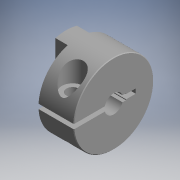
# Autodesk Inventor part: MCOCWK26-6_c
Saved by Autodesk Inventor 2017.3 (Build 213256000, 256)
## iProperties
Part Number: MCOCWK26-6_c
Material: Generic
Catalog Web Link: www.cadenas.de
Description: MCOC_coup-Couplings - Oldham Clamping Type
Vendor: MISUMI
Document SubType Name: Modeling
Designer: partserver
Manufacturer: MISUMI
Mass: 5.59398 g
Surface Area: 28.1267 cm^2
Volume: 5.59398 cm^3
Density: 1 g/cm^3
Appearance: PSOLRGB-192-192-192
Category: PARTsolutions
Company: MISUMI
Title: MCOCWK26-6
Author: Cadenas PARTsolutions
Comments: Couplings - Oldham Clamping Type
PSOL_IDENT_0: {$CADENAS_DATA\23d-libs\misumi\metric\50_couplings\mcoc\mcoc_coup.prj},208 {VTYP=3D},{NB=MCOCWK26-6_
PSOL_IDENT_1: c},{LINA=MCOCWK26-6},{NN=MCOC_coup},{DATE=30.03.2018 07:24:20},{GEOMDATE=05.12.2013 00:00:00},{VERSI
PSOL_IDENT_2: ON=},{LINEID=30},{WBVAR=HS,KGHS,ALT1,LDC,ALT2,RDC,DD,KGWC},{WBNUMERIC=LDC,RDC,DD}  {NB=MCOCWK26-6_c}
PSOL_IDENT_3: ,{LINA=MCOCWK26-6},{KT=DUMMY},{PN=MCOCWK26-6},{HS=},{KGHS=MCOCWK},{KGHSALG='MCOCLK','d1 (One Side)','
PSOL_IDENT_4: MCOCRK','d2 (One Side)','MCOCWK','d1*d2 (Both Sides)'},{MATH=304 Stainless Steel Sintered Alloy},{MA
PSOL_IDENT_5: TS=Carbon Reinforced Resin},{AC=Hexagon Socket Head Cap Screw},{TYPE=MCOCWK},{NO=26},{ALT1=},{ALT1AL
PSOL_IDENT_6: G=},{ALT13D=6},{DLALT1=6},{LDC=0.00},{LDCMIN=6},{LDCALG=0},{ALT2=},{ALT2ALG=},{ALT2ALG1= '', 'w/o RD
PSOL_IDENT_7: C (Shaft Hole Diameter Right Shaft)','RDC','with RDC (Shaft Hole Diameter Right Shaft)'},{ALT23D=6},
PSOL_IDENT_8: {RDC=0.00},{RDCALG=[0]},{DD=6.00},{DDALG=6,6.35,7,8,9.53,10,11,12},{DDPN=-6},{D=26.0},{D1=27},{D2=29
PSOL_IDENT_9: },{DD3=12.0},{L=30.4},{LL=11.5},{A=8.4},{F=5.0},{M=M4},{T=3.0},{ALTALG2='','Select RDC'},{HSALG='MCO
PSOL_IDENT_10: C','Standard Hole','','Key Groove Hole'},{TSIMD=4},{R1=7},{SC1=5.000},{SC2=5.000},{B=5.400},{L9=1.20
PSOL_IDENT_11: 0},{W=7.000},{G=4.000},{TT=1},{BB=2},{HSX=MCOCXK},{Z=7.155},{Z1=1.500},{KGWC=},{KGWCALG= '' , 'N/A'
PSOL_IDENT_12: },{KGWCPN=},{KGWC1=0},{TTKGW=0.0},{CIF=1},{BL=12}
NB: MCOCWK26-6_c
NN: MCOC_coup
NT: Couplings - Oldham Clamping Type
NBSYN: $PN._c
LINA: MCOCWK26-6
CATALOG: Misumi
PN: MCOCWK26-6
HS: Key Groove Hole
KGHS: d1*d2 (Both Sides)
NO: 26
ALT1: w/o LDC (Shaft Hole Diameter Left Shaft)
LDC: 0
ALT2: w/o RDC (Shaft Hole Diameter Right Shaft)
RDC: 0
DD: 6
D: 26
D1: 27
D2: 29
DD3: 12
L: 30.4
LL: 11.5
A: 8.4
F: 5
M: M4
T: 3.0
KGWC: N/A
SUPPLIER: MISUMI
ARTICLENO: MCOCWK26-6_c
BOMINFO: MCOCWK26-6
CREATOR: CADENAS GmbH
Autodesk Inventor part; units mm, degrees
sketch "Sketch_1" plane through (0, 0, 0) normal (0, 0, 1) x (1, 0, 0)
  line L0 (15.5, 0) -> (0, 0)
  line L1 (0, 0) -> (0, 12.8)
  line L2 (0, 12.8) -> (0.2, 13)
  line L3 (0.2, 13) -> (15.5, 13)
  line L4 (15.5, 13) -> (15.5, 0)
  line L5 (15.5, 0) -> (0, 0)
  constraints: 12 end point
revolve "Revolution1" add sketch "Sketch_1" angle 360 about axis through (15.5, 0, 0) along (1, 0, 0)
sketch "Sketch_6" plane through (0, 0, 0) normal (1, 0, 0) x (0, 1, 0)
  line L0 (-13, 0.75) -> (-13, -0.75)
  line L1 (-13, -0.75) -> (0, -0.75)
  line L2 (0, -0.75) -> (0, 0.75)
  line L3 (0, 0.75) -> (-13, 0.75)
  constraints: 8 end point
extrude "Extrusion1" cut sketch "Sketch_6" along normal blind 11.5
sketch "Sketch_7" plane through (5, 0, 0) normal (1, 0, 0) x (0, 0, -1)
  line L0 (-13, -8.4) -> (13, -8.4)
  line L1 (13, -8.4) -> (13, -11.9)
  line L2 (13, -11.9) -> (5, -11.9)
  line L3 (5, -11.9) -> (5, -10.4)
  line L4 (5, -10.4) -> (0.75, -10.4)
  line L5 (0.75, -10.4) -> (0.75, -8.4)
  line L6 (0.75, -8.4) -> (13, -8.4)
  constraints: 14 end point
revolve "Revolution2" cut sketch "Sketch_7" angle 360 about axis through (5, -8.4, 13) along (0, 0, 1)
sketch "Sketch4" plane through (11.5, 0, 0.75) normal (0, 0, -1) x (-1, 0, 0)
  point P0 (6.5, -8.4)
hole "Hole1" at (5, -8.4, 0.75) direction (0, 0, 1) diameter 3.242 depth 12.25 thread size "M4x0.7" class "6H" standard "ISO Metric profile"
sketch "Sketch_2" plane through (15.5, 0, 0) normal (1, 0, 0) x (0, 0, -1)
  line L0 (-14, -13.5) -> (14, -13.5)
  line L1 (14, -13.5) -> (14, 13.5)
  line L2 (14, 13.5) -> (-14, 13.5)
  line L3 (-14, 13.5) -> (-14, -13.5)
  line L4 (-13, -3.5) -> (13, -3.5)
  line L5 (13, -3.5) -> (13, 3.5)
  line L6 (13, 3.5) -> (-13, 3.5)
  line L7 (-13, 3.5) -> (-13, -3.5)
  constraints: 16 end point
extrude "Extrusion2" cut sketch "Sketch_2" against normal blind 4
sketch "Sketch6" plane through (15.5, 0, 0) normal (1, 0, 0) x (0, 0, -1)
  point P0 (0, 0)
hole "Hole2" at (15.5, 0, 0) direction (-1, 0, 0) diameter 13 depth 4
sketch "Sketch_15" plane through (11.5, 0, 0) normal (1, 0, 0) x (0, 0, -1)
  arc A0 (-1, 2.8284) -> (1, 2.8284) centre (0, 0) ccw
  line L0 (1, 2.8284) -> (1, 4)
  line L1 (1, 4) -> (-1, 4)
  line L2 (-1, 4) -> (-1, 2.8284)
  constraints: 6 end point, 2 point on circle, 1 centre point
extrude "Extrusion3" cut sketch "Sketch_15" along normal mid plane 31
sketch "Sketch_8" plane through (0, 0, 0) normal (1, 0, 0) x (0, 1, 0)
  line L0 (7.155, 0.75) -> (0, 0.75)
  line L1 (0, 0.75) -> (0, -0.75)
  line L2 (0, -0.75) -> (7.155, -0.75)
  line L3 (7.155, -0.75) -> (7.155, 0.75)
  constraints: 8 end point
extrude "Extrusion4" cut sketch "Sketch_8" along normal blind 15.5
ref_plane "L_XY" through (15.2, 0, 0) normal (1, 0, 0) x (0, 0, -1)
ref_plane "L_YZ" through (15.2, 0, 0) normal (0, 0, -1) x (0, 1, 0)
ref_plane "L_ZX" through (15.2, 0, 0) normal (0, 1, 0) x (1, 0, 0)
ref_plane "screw_XY" through (5, -8.4, -5) normal (0, 0, -1) x (1, 0, 0)
ref_plane "screw_YZ" through (5, -8.4, -5) normal (1, 0, 0) x (0, -1, 0)
ref_plane "screw_ZX" through (5, -8.4, -5) normal (0, -1, 0) x (0, 0, -1)
body "Solid1"
